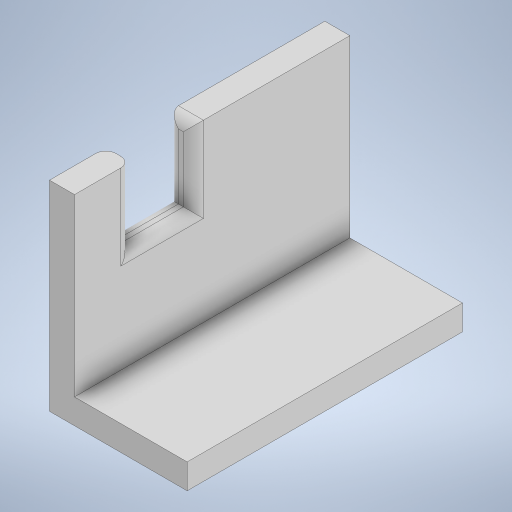
# Autodesk Inventor part: housing_mate_v09
Saved by Autodesk Inventor 2023 (Build 270158000, 158)
## iProperties
Created: 2023-11-20
Part Number: housing_mate_v09
Material: Generic
Document SubType Name: Modeling
Designer: Akramilab
Density: 1 g/cm^3
Appearance: Default
Author: Akramilab
Autodesk Inventor part; units mm, degrees
ref_plane "YZ Plane" through (0, 0, 0) normal (1, 0, 0) x (0, 1, 0)
ref_plane "XZ Plane" through (0, 0, 0) normal (0, 1, 0) x (-1, 0, 0)
ref_plane "XY Plane" through (0, 0, 0) normal (0, 0, 1) x (1, 0, 0)
sketch "Sketch1" plane through (0, 0, 0) normal (0, 0, 1) x (1, 0, 0)
  line L0 (0, 0) -> (2, 0)
  line L1 (2, 0) -> (2, 16)
  line L2 (2, 16) -> (0, 16)
  line L3 (0, 16) -> (0, 0)
  line L4 (2, 2) -> (11, 2)
  line L5 (11, 2) -> (11, 0)
  line L6 (11, 0) -> (2, 0)
  line L7 (2, 0) -> (2, 2)
  dimension "d0" = 2
  dimension "d1" = 16
  dimension "d2" = 9
  constraints: 16 end point, 4 parallel, 2 horizontal, 2 perpendicular, 1 point on line
  measures "d0" distance of L2.end L1.end
  measures "d1" distance of L1.end L0.end
  measures "d2" distance of L5.end L6.end
extrude "Extrusion1" add sketch "Sketch1" against normal blind 22
sketch "Sketch3" plane through (2, 2, 0) normal (1, 0, 0) x (0, 0, -1)
  line L0 (9.5, 14) -> (4.5, 14)
  line L1 (4.5, 14) -> (4.5, 8)
  line L2 (4.5, 8) -> (9.5, 8)
  line L3 (9.5, 8) -> (9.5, 14)
  point P0 (0, -2)
  dimension "d9" = 5
  dimension "d10" = 6
  constraints: 8 end point, 2 parallel, 1 horizontal, 1 perpendicular
  measures "d9" distance of L2.end L1.end
  measures "d10" distance of L1.end L0.end
extrude "Extrusion3" cut sketch "Sketch3" against normal blind 10
fillet "Fillet1" radius 0.8 7 edges at (2, 10, -7) (0, 10, -7) (1, 16, -9.5) (2, 13, -9.5) (0, 13, -9.5) (2, 13, -4.5) (0, 13, -4.5)
body "Solid1"
